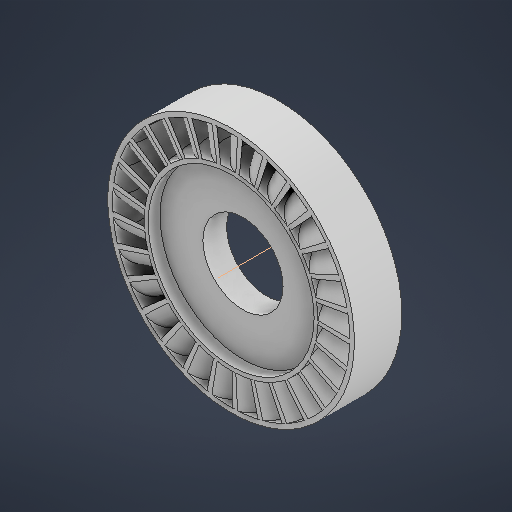
# Autodesk Inventor part: Palton 2
Saved by Autodesk Inventor 2025.3 (Build 293356030, 356C)
## iProperties
Created: 2025-09-16
Part Number: Palton 2
Material: Generic
Document SubType Name: Modeling
Designer: yo
Density: 1 g/cm^3
Appearance: Default
Author: yo
Autodesk Inventor part; units mm, degrees
ref_plane "YZ Plane" through (0, 0, 0) normal (1, 0, 0) x (0, 1, 0)
ref_plane "XZ Plane" through (0, 0, 0) normal (0, 1, 0) x (-1, 0, 0)
ref_plane "XY Plane" through (0, 0, 0) normal (0, 0, 1) x (1, 0, 0)
sketch "Sketch1" plane through (0, 0, 0) normal (0, 0, 1) x (1, 0, 0)
  circle A0 centre (0, 0) radius 18.3
  circle A1 centre (0, 0) radius 25
  circle A2 centre (0, 0) radius 17.5
  circle A3 centre (0, 0) radius 26
  dimension "d0" = 36.6
  dimension "d1" = 50
  dimension "d14" = 35
  dimension "d15" = 52
  constraints: 4 centre point, 4 coincident
  measures "d0" diameter of A0
  measures "d1" diameter of A1
  measures "d14" diameter of A2
  measures "d15" diameter of A3
extrude "Extrusion1" add sketch "Sketch1" along normal mid plane 5 contours A0 | A2
extrude "Extrusion2" add sketch "Sketch1" along normal mid plane 10 contours A1
sketch "Sketch2" plane through (0, 0, 5) normal (0, 0, 1) x (1, 0, 0)
  circle A0 centre (0, 0) radius 18.3 projected
  line L0 (18.3, 0) -> (25, 0)
  circle A1 centre (0, 0) radius 25 projected
  line L1 (18.022, 3.1778) -> (24.6202, 4.3412)
  dimension "d6" = 10
  constraints: 4 end point, 4 line through centre, 4 point on circle, 1 horizontal
  measures "d6" angle of L0 L1
sketch "Sketch7" plane through (0, 0, 0) normal (1, 0, 0) x (0, 1, 0)
  arc A0 (0, -5) -> (0, 5) centre (-1, 0) ccw
  line L0 (18.3, -5) -> (-18.3, -5) projected
  line L1 (-18.3, 5) -> (18.3, 5) projected
  point P0 (0, 0)
  dimension "d10" = 1
  constraints: 2 midpoint, 2 point on circle, 1 centre point, 1 horizontal alignment, 1 vertical alignment
  measures "d10" distance of A0.centre point (0, 0)
sweep "Sweep1" cut profiles "Sketch2" path "Sketch7" keep normal constant yes picked at (22.7526, 0.4845) path curves A0 contours A0 L1 A1 L0
pattern_circular "Circular Pattern1" count 29 over 360 about axis through (0, 0, 0) along (0, 0, 1) of "Sweep1"
extrude "Extrusion3" add sketch "Sketch1" along normal mid plane 10 contours A3
extrude "Extrusion4" add sketch "Sketch1" along normal mid plane 10 contours A0
sketch "Sketch8" plane through (0, 0, -2.5) normal (0, 0, -1) x (-1, 0, 0)
  circle A0 centre (0, 0) radius 8.45
  dimension "d20" = 16.9
  constraints: 1 centre point, 1 coincident
  measures "d20" diameter of A0
extrude "Extrusion5" cut sketch "Sketch8" against normal through all
body "Solid1"
